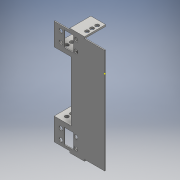
# Autodesk Inventor part: brace
Saved by Autodesk Inventor 2016 (Build 200138000, 138)
## iProperties
Created: 2016-02-21
Part Number: brace
Material: Generic
Document SubType Name: Modeling
Designer: mkepler
Density: 1 g/cm^3
Appearance: Default
Author: mkepler
Autodesk Inventor part; units mm, degrees
ref_plane "YZ Plane" through (0, 0, 0) normal (1, 0, 0) x (0, 1, 0)
ref_plane "XZ Plane" through (0, 0, 0) normal (0, 1, 0) x (-1, 0, 0)
ref_plane "XY Plane" through (0, 0, 0) normal (0, 0, 1) x (1, 0, 0)
sketch "Sketch1" plane through (0, 0, 0) normal (0, 1, 0) x (-1, 0, 0)
  line L0 (0, 0) -> (60, 0)
  line L1 (60, 0) -> (60, -24)
  line L2 (60, -24) -> (40, -24)
  line L3 (40, -24) -> (40, -100)
  line L4 (40, -100) -> (60, -100)
  line L5 (60, -100) -> (60, -124)
  line L6 (60, -124) -> (0, -124)
  line L7 (0, -124) -> (0, 0)
  dimension "d0" = 60
  dimension "d1" = 24
  dimension "d2" = 20
  dimension "d3" = 76
  dimension "d4" = 20
  dimension "d5" = 24
  constraints: 16 end point, 6 perpendicular, 1 horizontal, 1 vertical
  measures "d0" distance of L0.start L0.end
  measures "d1" distance of L0.end L1.end
  measures "d2" distance of L1.end L2.end
  measures "d3" distance of L2.end L3.end
  measures "d4" distance of L3.end L4.end
  measures "d5" distance of L4.end L5.end
extrude "Extrusion1" add sketch "Sketch1" along normal blind 1
sketch "Sketch2" plane through (0, 1, 0) normal (0, 1, 0) x (1, 0, 0)
  circle A0 centre (-52, 6) radius 2.2
  line L0 (-60, 0) -> (0, 0) projected
  line L1 (-60, 24) -> (-60, 0) projected
  circle A1 centre (-52, 18) radius 2.2
  line L2 (-48.25, 3) -> (-37.25, 3)
  line L3 (-37.25, 3) -> (-37.25, 21)
  line L4 (-37.25, 21) -> (-48.25, 21)
  line L5 (-48.25, 21) -> (-48.25, 3)
  circle A2 centre (-34, 17.9998) radius 2.2
  circle A3 centre (-33.9323, 6) radius 2.2
  line L6 (-40, 100) -> (-40, 24) projected
  line L7 (-40, 62) -> (0, 62)
  circle A4 centre (-52, 118) radius 2.2
  circle A5 centre (-52, 106) radius 2.2
  line L8 (-48.25, 121) -> (-37.25, 121)
  line L9 (-37.25, 121) -> (-37.25, 103)
  line L10 (-37.25, 103) -> (-48.25, 103)
  line L11 (-48.25, 103) -> (-48.25, 121)
  circle A6 centre (-34, 106.0002) radius 2.2
  circle A7 centre (-33.9323, 118) radius 2.2
  line L12 (-60, 124) -> (0, 124) projected
  line L13 (-60, 124) -> (-60, 100) projected
  dimension "d8" = 4.4
  dimension "d9" = 6
  dimension "d10" = 8
  dimension "d11" = 4.4
  dimension "d12" = 12
  dimension "d13" = 11
  dimension "d14" = 18
  dimension "d15" = 3
  dimension "d16" = 3.75
  dimension "d17" = 4.4
  dimension "d18" = 3.25
  dimension "d19" = 4.4
  dimension "d20" = 6
  dimension "d21" = 8
  dimension "d22" = 8
  constraints: 18 end point, 8 centre point, 8 symmetric about line, 2 horizontal, 2 parallel, 1 midpoint, 1 perpendicular, 4 other
  measures "d8" diameter of A0
  measures "d9" distance from line of L0 A0.centre
  measures "d10" distance from line of A0.centre L1
  measures "d11" diameter of A1
  measures "d12" distance of A1.centre A0.centre
  measures "d13" distance of L4.end L3.end
  measures "d14" distance of L3.end L2.end
  measures "d15" distance between parallel lines of L2 L0
  measures "d16" distance from line of L5 A1.centre
  measures "d17" diameter of A2
  measures "d18" distance from line of A2.centre L3
  measures "d19" diameter of A3
  measures "d20" distance from line of L12 A4.centre
  measures "d21" distance from line of L13 A5.centre
  measures "d22" distance from line of L13 A4.centre
extrude "Extrusion2" cut sketch "Sketch2" against normal blind 1.5
sketch "Sketch4" plane through (0, 1, 0) normal (0, 1, 0) x (1, 0, 0)
  line L0 (-60, 124) -> (-60, 100) projected
  line L1 (-60, 100) -> (-60, 97.5)
  line L2 (-60, 97.5) -> (-40, 97.5)
  line L3 (-40, 100) -> (-40, 24) projected
  line L4 (-40, 24) -> (-60, 24) projected
  line L5 (-60, 24) -> (-60, 26.5)
  line L6 (-60, 26.5) -> (-40, 26.5)
  line L7 (-40, 100) -> (-60, 100) projected
  line L8 (-40, 24) -> (-40, 100) projected
  line L9 (-60, 100) -> (-40, 100)
  line L10 (-40, 100) -> (-40, 97.5)
  line L11 (-60, 24) -> (-40, 24)
  line L12 (-40, 26.5) -> (-40, 24)
  line L13 (-60, 124) -> (-41.5, 124)
  line L14 (0, 124) -> (-60, 124) projected
  line L15 (-41.5, 124) -> (-41.5, 126)
  line L16 (-41.5, 126) -> (-24, 126)
  line L17 (-24, 126) -> (-24, 124)
  line L18 (-41.5, 124) -> (-24, 124)
  line L19 (-40, 62) -> (-22.3006, 62)
  line L20 (0, 0) -> (-60, 0)
  line L21 (-41.5, 0) -> (-41.5, -2)
  line L22 (-41.5, -2) -> (-24, -2)
  line L23 (-24, -2) -> (-24, 0)
  line L24 (-60, 0) -> (0, 0) projected
  dimension "d29" = 2.5
  dimension "d30" = 2.5
  dimension "d32" = 18.5
  dimension "d33" = 2
  dimension "d34" = 17.5
  constraints: 36 end point, 6 perpendicular, 6 point on line, 6 symmetric about line, 3 horizontal, 3 vertical, 2 collinear, 1 midpoint
  measures "d29" distance of L0.end L1.end
  measures "d30" distance of L4.end L5.end
  measures "d32" distance of L0.start L13.end
  measures "d33" distance of L13.end L15.end
  measures "d34" distance of L15.end L16.end
extrude "Extrusion3" add sketch "Sketch4" along normal blind 24 and the other way blind 1
sketch "Sketch6" plane through (-24, 25, -126) normal (0, 0, -1) x (-1, 0, 0)
  circle A0 centre (4, -6) radius 2.2
  line L0 (0, -25) -> (0, 0) projected
  line L1 (0, 0) -> (17.5, 0) projected
  circle A1 centre (4, -12) radius 2.2
  circle A2 centre (4, -18) radius 2.2
  line L2 (0, 0) -> (0, -24) projected
  line L3 (17.5003, -24) -> (0, -24)
  point P0 (-24, -25)
  dimension "d39" = 4.4
  dimension "d40" = 4
  dimension "d41" = 6
  dimension "d42" = 4.4
  dimension "d43" = 4.4
  dimension "d44" = 6
  dimension "d45" = 6
  dimension "d46" = 6
  constraints: 3 centre point, 2 end point, 1 horizontal
  measures "d39" diameter of A0
  measures "d40" distance from line of A0.centre L0
  measures "d41" distance from line of A0.centre L1
  measures "d42" diameter of A1
  measures "d43" diameter of A2
  measures "d44" distance of A0.centre A1.centre
  measures "d45" distance of A1.centre A2.centre
  measures "d46" distance from line of A2.centre L3
hole "Hole1" at (-28, 7, -126) at (-28, 13, -126) at (-28, 19, -126) direction (0, 0, 1) diameter 4.4 depth 2
sketch "Sketch7" plane through (-41.5, 25, 2) normal (0, 0, 1) x (1, 0, 0)
  line L0 (17.5, -24) -> (0, -24) projected
  line L1 (0, -24) -> (0, -25) projected
  line L2 (17.5, -24) -> (0, -24)
  circle A0 centre (13.5, -18) radius 2.2 projected
  circle A1 centre (13.5, -18) radius 2.2
  circle A2 centre (13.5, -12) radius 2.2 projected
  circle A3 centre (13.5, -12) radius 2.2
  circle A4 centre (13.5, -6) radius 2.2 projected
  circle A5 centre (13.5, -6) radius 2.2
  point P0 (41.5, -25)
  dimension "d54" = 4.4
  dimension "d55" = 4.4
  dimension "d56" = 4.4
  constraints: 3 centre point, 3 coincident, 2 end point, 1 horizontal
  measures "d54" diameter of A1
  measures "d55" diameter of A3
  measures "d56" diameter of A5
hole "Hole2" at (-28, 7, 2) at (-28, 13, 2) at (-28, 19, 2) direction (0, 0, -1) diameter 4.4 depth 2
sketch "Sketch11" plane through (-60, 1, -100) normal (0, 0, -1) x (-1, 0, 0)
  circle A0 centre (-8, 18) radius 2.2
  line L0 (0, 24) -> (0, 0) projected
  line L1 (-20, 24) -> (0, 24) projected
  circle A1 centre (-8, 12) radius 2.2
  circle A2 centre (-8, 6) radius 2.2
  circle A3 centre (-31.5, 6) radius 2.2
  circle A4 centre (-31.5, 12) radius 2.2
  circle A5 centre (-31.5, 18) radius 2.2
  point P0 (-60, -1)
  point P1 (-36, 24)
  dimension "d68" = 4.4
  dimension "d69" = 8
  dimension "d70" = 6
  dimension "d71" = 4.4
  dimension "d72" = 4.4
  dimension "d73" = 6
  dimension "d74" = 6
  dimension "d82" = 4.4
  dimension "d83" = 23.5
  dimension "d84" = 4.4
  dimension "d85" = 4.4
  constraints: 6 centre point
  measures "d68" diameter of A0
  measures "d69" distance from line of A0.centre L0
  measures "d70" distance from line of L1 A0.centre
  measures "d71" diameter of A1
  measures "d72" diameter of A2
  measures "d73" distance of A1.centre A0.centre
  measures "d74" distance of A2.centre A1.centre
  measures "d82" diameter of A3
  measures "d83" distance of A3.centre A2.centre
  measures "d84" diameter of A4
  measures "d85" diameter of A5
hole "Hole3" at (-52, 19, -100) at (-52, 13, -100) at (-52, 7, -100) direction (0, 0, 1) diameter 4.4 depth 2.5
sketch "Sketch12" plane through (-60, 1, -24) normal (0, 0, 1) x (1, 0, 0)
  circle A0 centre (8, 6) radius 2.2 projected
  circle A1 centre (8, 6) radius 2.2
  circle A2 centre (8, 12) radius 2.2 projected
  circle A3 centre (8, 12) radius 2.2
  circle A4 centre (8, 18) radius 2.2 projected
  circle A5 centre (8, 18) radius 2.2
  point P0 (60, -1)
  dimension "d86" = 4.4
  dimension "d87" = 4.4
  dimension "d88" = 4.4
  constraints: 3 centre point, 3 coincident
  measures "d86" diameter of A1
  measures "d87" diameter of A3
  measures "d88" diameter of A5
hole "Hole4" at (-52, 7, -24) at (-52, 13, -24) at (-52, 19, -24) direction (0, 0, -1) diameter 4.4 depth 2.5
sketch "Sketch13" plane through (-60, 1, -24) normal (0, 0, 1) x (1, 0, 0)
  point P0 (60, -1)
body "Solid1"
